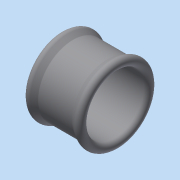
# Autodesk Inventor part: Обмотка статора
Saved by Autodesk Inventor 2016 SP1 (Build 200210100, 210)
## iProperties
Created: 2016-05-17
Part Number: Обмотка статора
Material: Медь
Document SubType Name: Modeling
Designer: a.kaluzhenin
Density: 8.94 g/cm^3
Appearance: Медь - сатинированная
Author: a.kaluzhenin
Autodesk Inventor part; units mm, degrees
ref_plane "YZ Plane" through (0, 0, 0) normal (1, 0, 0) x (0, 1, 0)
ref_plane "XZ Plane" through (0, 0, 0) normal (0, 1, 0) x (-1, 0, 0)
ref_plane "XY Plane" through (0, 0, 0) normal (0, 0, 1) x (1, 0, 0)
sketch "Эскиз1" plane through (0, 0, 0) normal (0, 0, 1) x (1, 0, 0)
  line L0 (-235.1726, -42.1752) -> (-170.2444, -42.1752)
  line L1 (-249.7085, -52.574) -> (-155.7085, -52.574)
  line L2 (-169.2444, -41.9072) -> (-159.7085, -36.4017)
  arc A0 (-155.7085, -52.574) -> (-159.7085, -36.4017) centre (-155.7085, -43.9932) ccw
  line L3 (-202.7085, -52.574) -> (-202.7085, -42.1752) construction
  line L4 (-236.1726, -41.9072) -> (-245.7085, -36.4017)
  arc A1 (-245.7085, -36.4017) -> (-249.7085, -52.574) centre (-249.7085, -43.9932) ccw
  arc A2 (-236.1726, -41.9072) -> (-235.1726, -42.1752) centre (-235.1726, -40.1752) ccw
  arc A3 (-170.2444, -42.1752) -> (-169.2444, -41.9072) centre (-170.2444, -40.1752) ccw
  line L5 (-312.1183, 0) -> (52.0197, 0) projected
  point P0 (0, 0)
  point P1 (-235.7085, -42.1752)
  point P2 (-169.7085, -42.1752)
  point P3 (-147.1302, -43.7828)
  dimension "d0" = 66
  dimension "d1" = 94
  dimension "d2" = 30
  dimension "d3" = 10
  dimension "d4" = 2
  dimension "d5" = 2
  constraints: 10 end point, 9 point on circle, 4 centre point, 4 point on line, 4 tangent, 2 coincident, 2 horizontal, 2 midpoint, 2 symmetric about line, 1 perpendicular, 1 vertical alignment, 1 other
  measures "d0" distance of point (-169.708, -42.175) point (-235.708, -42.175)
  measures "d1" distance of L1.start L1.end
  measures "d2" angle of L2 L0
  measures "d3" horizontal distance of L2.end point (-169.708, -42.175)
  measures "d4" radius of A2
  measures "d5" radius of A3
revolve "Вращение1" add sketch "Эскиз1" angle 360 about axis through (-10, 0, 0) along (1, 0, 0)
